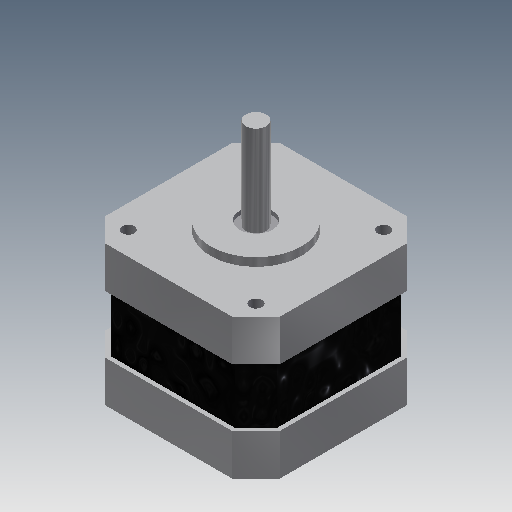
# Autodesk Inventor part: Motor_paso
Saved by Autodesk Inventor 2018 (Build 220112000, 112)
## iProperties
Created: 2018-10-12
Part Number: Motor_paso
Material: Generic
Document SubType Name: Modeling
Designer: Emily
Density: 1 g/cm^3
Appearance: Default
Author: Emily
Autodesk Inventor part; units mm, degrees
ref_plane "YZ Plane" through (0, 0, 0) normal (1, 0, 0) x (0, 1, 0)
ref_plane "XZ Plane" through (0, 0, 0) normal (0, 1, 0) x (-1, 0, 0)
ref_plane "XY Plane" through (0, 0, 0) normal (0, 0, 1) x (1, 0, 0)
sketch "Sketch2" plane through (0, 0, 0) normal (0, 1, 0) x (-1, 0, 0)
  line L0 (15, 20.15) -> (20.15, 15)
  line L1 (20.15, 15) -> (20.15, -15)
  line L2 (20.15, -15) -> (15, -20.15)
  line L3 (15, -20.15) -> (-15, -20.15)
  line L4 (-15, -20.15) -> (-20.15, -15)
  line L5 (-20.15, -15) -> (-20.15, 15)
  line L6 (-20.15, 15) -> (-15, 20.15)
  line L7 (-15, 20.15) -> (15, 20.15)
  point P0 (0, 0)
  point P1 (20.15, 0)
  point P2 (0, -20.15)
  dimension "d2" = 30
  dimension "d3" = 40.3
  dimension "d4" = 135
  constraints: 16 end point, 6 perpendicular, 3 horizontal alignment, 3 vertical alignment, 2 midpoint, 1 vertical
  measures "d2" distance of L2.end L3.end
  measures "d3" distance of L2.end L0.start
  measures "d4" angle of L2 L1
extrude "Extrusion1" add sketch "Sketch2" along normal mid plane 34
sketch "Sketch7" plane through (0, 17, 0) normal (0, 1, 0) x (1, 0, 0)
  circle A0 centre (0, 0) radius 11
  dimension "d27" = 22
  constraints: 1 centre point, 1 coincident
  measures "d27" diameter of A0
extrude "Extrusion3" add sketch "Sketch7" along normal blind 2
sketch "Sketch8" plane through (0, 19, 0) normal (0, 1, 0) x (1, 0, 0)
  circle A0 centre (0, 0) radius 4
  dimension "d30" = 8
  constraints: 1 centre point, 1 coincident
  measures "d30" diameter of A0
extrude "Extrusion4" cut sketch "Sketch8" against normal blind 1
sketch "Sketch9" plane through (0, 18, 0) normal (0, 1, 0) x (1, 0, 0)
  circle A0 centre (0, 0) radius 2.5
  dimension "d33" = 5
  constraints: 1 centre point, 1 coincident
  measures "d33" diameter of A0
extrude "Extrusion5" add sketch "Sketch9" along normal blind 22
sketch "Sketch10" plane through (-15, 17, 20.15) normal (0, 0, 1) x (1, 0, 0)
  line L0 (30, 0) -> (30, -34) projected
  line L1 (0, 0) -> (30, 0) projected
  line L2 (0, -34) -> (0, 0) projected
  line L3 (30, -34) -> (0, -34) projected
  line L4 (0, 0) -> (30, 0)
  line L5 (30, 0) -> (30, -10)
  line L6 (30, -10) -> (0, -10)
  line L7 (0, -10) -> (0, 0)
  line L8 (0, 0) -> (30, -10) construction
  line L9 (30, 0) -> (0, -10) construction
  line L10 (0, -24) -> (30, -24)
  line L11 (30, -24) -> (30, -34)
  line L12 (30, -34) -> (0, -34)
  line L13 (0, -34) -> (0, -24)
  line L14 (0, -24) -> (30, -34) construction
  line L15 (30, -24) -> (0, -34) construction
  line L16 (0, 0) -> (30, 0) projected
  point P0 (15, -17)
  point P1 (15, -5)
  point P2 (15, -29)
  dimension "d36" = 10
  dimension "d37" = 10
  constraints: 24 end point, 4 midpoint, 4 parallel, 2 equal length, 2 horizontal, 2 perpendicular
  measures "d36" distance of L0.start L5.end
  measures "d37" distance of L0.end L10.end
extrude "Extrusion6" add sketch "Sketch10" along normal blind 1 contours L0 L6 L2 L1 | L0 L3 L2 L10
mirror "Mirror1" about plane through (0, 0, 0) normal (0, 0, 1) of "Extrusion6"
sketch "Sketch11" plane through (20.15, -17, -15) normal (1, 0, 0) x (0, 0, -1)
  line L0 (0, 34) -> (0, 0) projected
  line L1 (-30, 34) -> (0, 34) projected
  line L2 (-30, 34) -> (-30, 0) projected
  line L3 (0, 0) -> (-30, 0) projected
  line L4 (-30, 34) -> (0, 34)
  line L5 (0, 34) -> (0, 24)
  line L6 (0, 24) -> (-30, 24)
  line L7 (-30, 24) -> (-30, 34)
  line L8 (-30, 34) -> (0, 24) construction
  line L9 (0, 34) -> (-30, 24) construction
  line L10 (-30, 10) -> (0, 10)
  line L11 (0, 10) -> (0, 0)
  line L12 (0, 0) -> (-30, 0)
  line L13 (-30, 0) -> (-30, 10)
  line L14 (-30, 10) -> (0, 0) construction
  line L15 (0, 10) -> (-30, 0) construction
  line L16 (-30, 34) -> (0, 34) projected
  point P0 (-15, 17)
  point P1 (-15, 29)
  point P2 (-15, 5)
  dimension "d40" = 10
  constraints: 24 end point, 4 midpoint, 4 parallel, 3 equal length, 2 horizontal, 2 perpendicular
  measures "d40" distance of L0.start L5.end
extrude "Extrusion7" add sketch "Sketch11" along normal blind 1 contours L0 L6 L2 L1 | L0 L3 L2 L10
mirror "Mirror2" about plane through (0, 0, 0) normal (1, 0, 0) of "Extrusion7"
sketch "Sketch12" plane through (-15, -7, 20.15) normal (-0.7071, 0, 0.7071) x (0.7071, 0, 0.7071)
  line L0 (0, -10) -> (0, 0) projected
  line L1 (0, 0) -> (0, 14) projected
  line L2 (0, 14) -> (0, 24) projected
  line L3 (-7.2832, 24) -> (0, 24) projected
  line L4 (-7.2832, 24) -> (-7.2832, 14) projected
  line L5 (-7.2832, 14) -> (-7.2832, 0) projected
  line L6 (-7.2832, 0) -> (-7.2832, -10) projected
  line L7 (0, -10) -> (-7.2832, -10) projected
  line L8 (-7.2832, 24) -> (0, 24)
  line L9 (0, 24) -> (0, 14)
  line L10 (0, 14) -> (-7.2832, 14)
  line L11 (-7.2832, 14) -> (-7.2832, 24)
  line L12 (-7.2832, 24) -> (0, 14) construction
  line L13 (0, 24) -> (-7.2832, 14) construction
  line L14 (-7.2832, 0) -> (0, 0)
  line L15 (0, 0) -> (0, -10)
  line L16 (0, -10) -> (-7.2832, -10)
  line L17 (-7.2832, -10) -> (-7.2832, 0)
  line L18 (-7.2832, 0) -> (0, -10) construction
  line L19 (0, 0) -> (-7.2832, -10) construction
  line L20 (-7.2832, 24) -> (0, 24) projected
  line L21 (0, -10) -> (-7.2832, -10) projected
  point P0 (-3.6416, 7)
  point P1 (-3.6416, 19)
  point P2 (-3.6416, -5)
  dimension "d43" = 10
  dimension "d44" = 10
  constraints: 24 end point, 4 midpoint, 4 parallel, 2 collinear, 2 horizontal, 2 perpendicular
  measures "d43" distance of L6.end L14.start
  measures "d44" distance of L2.end L9.end
extrude "Extrusion8" add sketch "Sketch12" along normal blind 1 contours L7 L6 L14 L0 | L10 L4 L3 L2
sketch "Sketch14" plane through (-15, 7, 21.15) normal (-1, 0, 0) x (0, 0, 1)
  line L0 (-1, 0) -> (-1, 10) projected
  line L1 (-1, 0) -> (0, 0) projected
  line L2 (0, 10) -> (0, 0) projected
  line L3 (-1, 10) -> (0, 10) projected
  line L4 (-1, -24) -> (-1, -14) projected
  line L5 (-1, -24) -> (0, -24) projected
  line L6 (0, -14) -> (0, -24) projected
  line L7 (-1, -14) -> (0, -14) projected
  point P0 (-21.15, -7)
extrude "Extrusion9" add sketch "Sketch14" along normal up to surface surface through (-18.2821, 12, 18.2821) normal (-0.7071, 0, 0.7071)
sketch "Sketch15" plane through (-21.15, 7, 15) normal (0, 0, 1) x (1, 0, 0)
  line L0 (1, 10) -> (1, 0) projected
  line L1 (1, 10) -> (0, 10) projected
  line L2 (0, 10) -> (0, 0) projected
  line L3 (1, 0) -> (0, 0) projected
  line L4 (1, -14) -> (1, -24) projected
  line L5 (1, -14) -> (0, -14) projected
  line L6 (0, -14) -> (0, -24) projected
  line L7 (1, -24) -> (0, -24) projected
  point P0 (21.15, -7)
extrude "Extrusion10" add sketch "Sketch15" along normal up to surface surface through (-18.2821, -12, 18.2821) normal (-0.7071, 0, 0.7071)
mirror "Mirror3" about plane through (0, 0, 0) normal (1, 0, 0) of "Extrusion8", "Extrusion9", "Extrusion10"
mirror "Mirror4" about plane through (0, 0, 0) normal (0, 0, 1) of "Extrusion8", "Extrusion9", "Extrusion10", "Mirror3"
sketch "Sketch17" plane through (0, 17, 0) normal (0, 1, 0) x (1, 0, 0)
  line L0 (-21.15, -15.4142) -> (-15.4142, -21.15) projected
  line L1 (-15.4142, -21.15) -> (15.4142, -21.15) projected
  line L2 (21.15, -15.4142) -> (15.4142, -21.15) projected
  line L3 (21.15, -15.4142) -> (21.15, 15.4142) projected
  line L4 (21.15, 15.4142) -> (15.4142, 21.15) projected
  line L5 (15.4142, 21.15) -> (-15.4142, 21.15) projected
  line L6 (-21.15, 15.4142) -> (-15.4142, 21.15) projected
  line L7 (-21.15, 15.4142) -> (-21.15, -15.4142) projected
  circle A0 centre (0, 0) radius 11 projected
  circle A1 centre (-15.5, -15.5) radius 1.5
  circle A2 centre (-15.5, 15.5) radius 1.5
  circle A3 centre (15.5, 15.5) radius 1.5
  circle A4 centre (15.5, -15.5) radius 1.5
  dimension "d53" = 3
  dimension "d54" = 31
  dimension "d55" = 31
  dimension "d57" = 15.5
  dimension "d66" = 15.5
  constraints: 4 centre point, 3 equal radius, 2 horizontal alignment, 2 vertical alignment
  measures "d53" diameter of A1
  measures "d54" distance of A4.centre A1.centre
  measures "d55" distance of A1.centre A2.centre
  measures "d57" horizontal distance of A2.centre point (0, 0)
  measures "d66" horizontal distance of A1.centre point (0, 0)
hole "Hole3" at (-15.5, 17, 15.5) at (-15.5, 17, -15.5) at (15.5, 17, -15.5) at (15.5, 17, 15.5) direction (0, -1, 0) diameter 3 depth 4.5
ref_plane "Work Plane1" through (0, 0, 0) normal (1, 0, 0) x (0, 1, 0)
ref_plane "Work Plane2" through (0, 0, 0) normal (-1, 0, 0) x (0, 1, 0)
ref_plane "Work Plane3" through (0, 0, 0) normal (-1, 0, 0) x (0, 1, 0)
body "Solid1"
